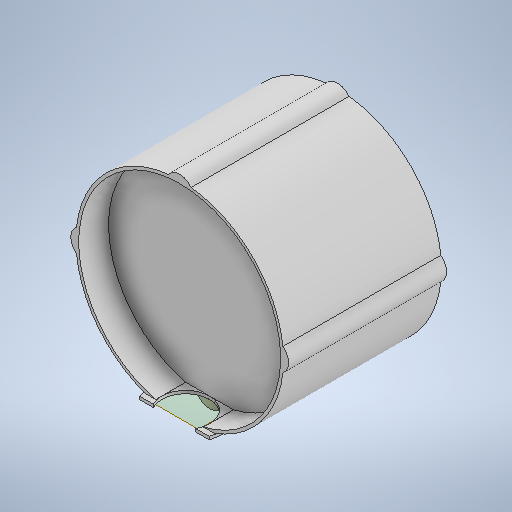
# Autodesk Inventor part: 2024_08_26_Double_walled_beaker_recess_2,1cm
Saved by Autodesk Inventor 2025.1 (Build 291241000, 241)
## iProperties
Created: 2023-11-21
Part Number: 2024_08_26_Double_walled_beaker_recess_2,1cm
Material: Generisch
Document SubType Name: Modeling
Designer: Daniel
Density: 1 g/cm^3
Appearance: Vorgabe
Author: Daniel
Autodesk Inventor part; units mm, degrees
ref_plane "YZ Plane" through (0, 0, 0) normal (1, 0, 0) x (0, 1, 0)
ref_plane "XZ Plane" through (0, 0, 0) normal (0, 1, 0) x (-1, 0, 0)
ref_plane "XY Plane" through (0, 0, 0) normal (0, 0, 1) x (1, 0, 0)
sketch "Sketch1" plane through (0, 0, 0) normal (0, 0, 1) x (1, 0, 0)
  circle A0 centre (0, 0) radius 11.25
  circle A1 centre (0, 0) radius 35.025
  circle A2 centre (0, 0) radius 37.030393
  arc A3 (-32.79294, -17.200962) -> (-31.29294, -19.799038) centre (0, 0) ccw
  line L0 (-32.79294, -17.200962) -> (-31.05471, -16.197395)
  line L1 (-32.79294, -17.200962) -> (-31.05471, -16.197395)
  line L2 (-29.55471, -18.795471) -> (-31.29294, -19.799038)
  line L3 (-31.29294, -19.799038) -> (-29.55471, -18.795471)
  line L4 (-16.197395, -31.05471) -> (-17.200962, -32.79294)
  line L5 (-17.200962, -32.79294) -> (-16.197395, -31.05471)
  arc A4 (-19.799038, -31.29294) -> (-17.200962, -32.79294) centre (0, 0) ccw
  line L6 (-19.799038, -31.29294) -> (-18.795471, -29.55471)
  line L7 (-19.799038, -31.29294) -> (-18.795471, -29.55471)
  arc A5 (17.200962, -32.79294) -> (19.799038, -31.29294) centre (0, 0) ccw
  line L8 (17.200962, -32.79294) -> (16.197395, -31.05471)
  line L9 (17.200962, -32.79294) -> (16.197395, -31.05471)
  line L10 (18.795471, -29.55471) -> (19.799038, -31.29294)
  line L11 (19.799038, -31.29294) -> (18.795471, -29.55471)
  arc A6 (31.29294, -19.799038) -> (32.79294, -17.200962) centre (0, 0) ccw
  line L12 (31.29294, -19.799038) -> (29.55471, -18.795471)
  line L13 (31.05471, -16.197395) -> (32.79294, -17.200962)
  line L14 (32.79294, -17.200962) -> (31.05471, -16.197395)
  line L15 (32.79294, 17.200962) -> (31.05471, 16.197395)
  line L16 (32.79294, 17.200962) -> (31.05471, 16.197395)
  arc A7 (32.79294, 17.200962) -> (31.29294, 19.799038) centre (0, 0) ccw
  line L17 (29.55471, 18.795471) -> (31.29294, 19.799038)
  line L18 (31.29294, 19.799038) -> (29.55471, 18.795471)
  line L19 (16.197395, 31.05471) -> (17.200962, 32.79294)
  line L20 (17.200962, 32.79294) -> (16.197395, 31.05471)
  line L21 (19.799038, 31.29294) -> (18.795471, 29.55471)
  line L22 (19.799038, 31.29294) -> (18.795471, 29.55471)
  line L23 (-17.200962, 32.79294) -> (-16.197395, 31.05471)
  line L24 (-17.200962, 32.79294) -> (-16.197395, 31.05471)
  line L25 (-18.795471, 29.55471) -> (-19.799038, 31.29294)
  line L26 (-19.799038, 31.29294) -> (-18.795471, 29.55471)
  arc A8 (-31.29294, 19.799038) -> (-32.79294, 17.200962) centre (0, 0) ccw
  line L27 (-31.29294, 19.799038) -> (-29.55471, 18.795471)
  line L28 (-31.29294, 19.799038) -> (-29.55471, 18.795471)
  line L29 (-31.05471, 16.197395) -> (-32.79294, 17.200962)
  line L30 (-32.79294, 17.200962) -> (-31.05471, 16.197395)
  arc A9 (-34.800207, -3.961848) -> (-34.800207, 3.961848) centre (-31.75, 0) ccw
  circle A10 centre (-31.75, 0) radius 5
  arc A11 (-3.961848, 34.800207) -> (3.961848, 34.800207) centre (0, 31.75) ccw
  circle A12 centre (0, 31.75) radius 5
  circle A13 centre (31.75, 0) radius 5
  circle A14 centre (31.75, 0) radius 5
  arc A15 (-3.961848, -34.800207) -> (3.961848, -34.800207) centre (0, -31.75) ccw
  circle A16 centre (0, -31.75) radius 5
  circle A17 centre (0, 31.75) radius 4.75
  circle A18 centre (-31.75, 0) radius 4.75
  circle A19 centre (0, -31.75) radius 4.75
  circle A20 centre (31.75, 0) radius 4.75
  circle A21 centre (0, 0) radius 34.775
  circle A22 centre (0, 0) radius 36.75
  point P0 (0, 0)
  point P1 (0, 49.75)
  point P2 (34.563789, -3.82689)
  point P3 (34.563789, 3.82689)
  point P4 (3.82689, 34.563789)
  point P5 (-3.82689, 34.563789)
  point P6 (-34.563789, 3.82689)
  point P7 (-34.563789, -3.82689)
  point P8 (-3.82689, -34.563789)
  point P9 (3.82689, -34.563789)
  dimension "d6" = 70.05
  dimension "d8" = 74.06079
  dimension "d0" = 10
  dimension "d1" = 0.25
  dimension "d4" = 360
  dimension "d7" = 0.25
  dimension "d9" = 73.5
  constraints: 62 end point, 21 centre point, 18 point on circle, 15 collinear, 10 coincident, 16 other
  measures "d0" diameter of A12
  measures "d1" radial gap between concentric circles of A12 A17
  measures "d9" diameter of A22
sketch "Sketch1 outline for Extrusion1" plane through (0, 0, 0) normal (0, 0, 1) x (1, 0, 0)
  arc A0 (3.82689, -34.563789) -> (34.563789, -3.82689) centre (0, 0) ccw
  arc A1 (-3.82689, -34.563789) -> (3.82689, -34.563789) centre (0, -31.75) ccw
  arc A2 (-34.563789, -3.82689) -> (-3.82689, -34.563789) centre (0, 0) ccw
  arc A3 (-34.563789, 3.82689) -> (-34.563789, -3.82689) centre (-31.75, 0) ccw
  arc A4 (-3.82689, 34.563789) -> (-34.563789, 3.82689) centre (0, 0) ccw
  arc A5 (3.82689, 34.563789) -> (-3.82689, 34.563789) centre (0, 31.75) ccw
  arc A6 (34.563789, 3.82689) -> (3.82689, 34.563789) centre (0, 0) ccw
  arc A7 (34.563789, -3.82689) -> (34.563789, 3.82689) centre (31.75, 0) ccw
extrude "Extrusion1" add sketch "Sketch1 outline for Extrusion1" along normal blind 52.9
sketch "Skizze4" plane through (0, 0, 52.9) normal (0, 0, 1) x (1, 0, 0)
  circle A0 centre (0, 0) radius 33.79
  dimension "d24" = 67.58
  constraints: 1 centre point, 1 coincident
  measures "d24" diameter of A0
extrude "Extrusion4" cut sketch "Skizze4" against normal blind 10
sketch "Skizze5" plane through (0, 0, 52.9) normal (0, 0, 1) x (1, 0, 0)
  line L0 (-8, -25.79) -> (8, -25.79)
  line L1 (8, -25.79) -> (8, -41.79)
  line L2 (8, -41.79) -> (-8, -41.79)
  line L3 (-8, -41.79) -> (-8, -25.79)
  circle A0 centre (0, 0) radius 33.79 projected
  line L4 (-8, -25.79) -> (8, -41.79) construction
  line L5 (8, -25.79) -> (-8, -41.79) construction
  point P0 (0, -33.79)
  dimension "d27" = 16
  dimension "d28" = 16
  constraints: 12 end point, 2 midpoint, 2 parallel, 1 horizontal, 1 perpendicular, 1 vertical alignment, 1 other
  measures "d27" distance of L1.end L2.end
  measures "d28" distance of L0.end L1.end
extrude "Extrusion5" cut sketch "Skizze5" against normal up to surface (10 mm away) contours L0 L1 A0 L3 | A0 L1 L2 L3 picked at (-0.896461, -28.420935)
ref_plane "Arbeitsebene1" through (-8, -33.84229, 52.9) normal (0, -1, 0) x (0, 0, -1)
sketch "Skizze8" plane through (-8, -33.84229, 52.9) normal (0, -1, 0) x (0, 0, -1)
  circle A0 centre (2, 8) radius 8
  circle A1 centre (2, 8) radius 12.247788
  line L0 (-1.778493, -7.044693) -> (-1.736571, 22.979568)
  line L1 (10, 0) -> (2, 0)
  line L2 (2, 0) -> (2, 8)
  line L3 (2, 8) -> (10, 8)
  line L4 (10, 8) -> (10, 0)
  point P0 (52.9, 8)
  point P1 (3.776106, -5.296677)
  point P2 (-1.741203, 19.662406)
  point P3 (-1.747618, 15.067911)
  point P4 (-1.76734, 0.942582)
  point P5 (-1.773756, -3.651913)
  dimension "d31" = 16
  dimension "d36" = 8
  constraints: 10 end point, 2 parallel, 1 centre point, 1 coincident, 1 horizontal, 1 perpendicular, 2 other
  measures "d31" diameter of A0
  measures "d36" distance of L2.end L3.end
extrude "Extrusion6" add sketch "Skizze8" against normal blind 1 contours L1 L4 A0 L0 A1 | A0 L4 L1
body "Solid1"
